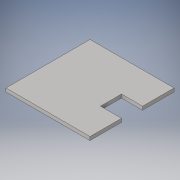
# Autodesk Inventor part: Bottom_chasis
Saved by Autodesk Inventor 2016 (Build 200138000, 138)
## iProperties
Created: 2016-02-28
Part Number: Bottom_chasis
Material: Generic
Document SubType Name: Modeling
Designer: torti_000
Density: 1 g/cm^3
Appearance: Default
Author: torti_000
Autodesk Inventor part; units mm, degrees
ref_plane "YZ Plane" through (0, 0, 0) normal (1, 0, 0) x (0, 1, 0)
ref_plane "XZ Plane" through (0, 0, 0) normal (0, 1, 0) x (-1, 0, 0)
ref_plane "XY Plane" through (0, 0, 0) normal (0, 0, 1) x (1, 0, 0)
sketch "Sketch1" plane through (0, 0, 0) normal (0, 1, 0) x (-1, 0, 0)
  line L0 (0, 0) -> (152.4, 0)
  line L1 (152.4, 0) -> (152.4, -152.4)
  line L2 (152.4, -152.4) -> (0, -152.4)
  line L3 (0, -152.4) -> (0, -101.6)
  line L4 (0, 0) -> (0, -50.8)
  line L5 (0, -50.8) -> (0, -57.15)
  line L6 (0, -101.6) -> (0, -95.25)
  line L7 (0, -57.15) -> (38.1, -57.15)
  line L8 (38.1, -57.15) -> (38.1, -95.25)
  line L9 (38.1, -95.25) -> (0, -95.25)
  dimension "d0" = 152.4
  dimension "d1" = 152.4
  dimension "d6" = 57.15
  dimension "d7" = 57.15
  dimension "d8" = 38.1
  constraints: 20 end point, 5 perpendicular, 3 vertical, 2 horizontal
  measures "d0" distance of L0.start L0.end
  measures "d1" distance of L0.end L1.end
  measures "d6" distance of L5.end L0.start
  measures "d7" distance of L2.end L6.end
  measures "d8" distance of L5.end L7.end
extrude "Extrusion1" add sketch "Sketch1" along normal blind 6.35
body "Solid1"
